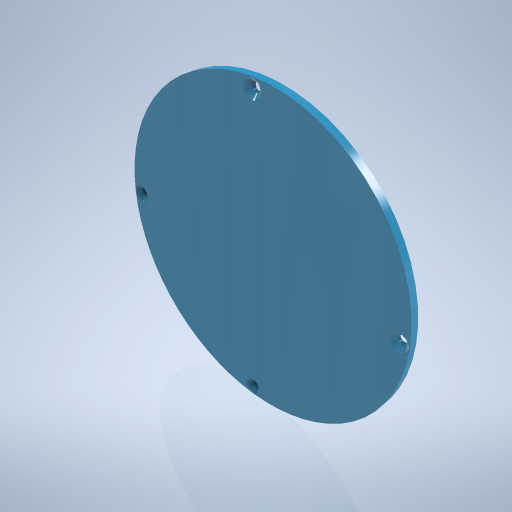
# Autodesk Inventor part: plate
Saved by Autodesk Inventor 2024.2 (Build 282272000, 272)
## iProperties
Created: 2024-04-01
Part Number: plate
Material: Gold
Document SubType Name: Modeling
Designer: Fabri
Density: 19.3 g/cm^3
Appearance: Himmelblau - dunkel
Author: Fabri
Autodesk Inventor part; units mm, degrees
ref_plane "YZ Plane" through (0, 0, 0) normal (1, 0, 0) x (0, 1, 0)
ref_plane "XZ Plane" through (0, 0, 0) normal (0, 1, 0) x (-1, 0, 0)
ref_plane "XY Plane" through (0, 0, 0) normal (0, 0, 1) x (1, 0, 0)
sketch "Skizze1" plane through (0, 0, 0) normal (0, 0, 1) x (1, 0, 0)
  line L0 (0, 0) -> (0, 15)
  line L1 (0, 2.5) -> (-9, 2.5)
  line L2 (-9, 2.5) -> (-9.567, 1.5179)
  arc A0 (-10.433, 1.5179) -> (-9.567, 1.5179) centre (-10, 1.7679) ccw
  line L3 (-10.433, 1.5179) -> (-11, 2.5)
  line L4 (-11, 2.5) -> (-12, 2.5)
  line L5 (-12, 2.5) -> (-12.567, 1.5179)
  arc A1 (-13.433, 1.5179) -> (-12.567, 1.5179) centre (-13, 1.7679) ccw
  line L6 (-13.433, 1.5179) -> (-14, 2.5)
  line L7 (-10, 1.7679) -> (-10, 5.291) construction
  line L8 (-14, 2.5) -> (-15, 2.5)
  line L9 (-15, 2.5) -> (-15.567, 1.5179)
  arc A2 (-16.433, 1.5179) -> (-15.567, 1.5179) centre (-16, 1.7679) ccw
  line L10 (-16.433, 1.5179) -> (-17, 2.5)
  line L11 (-17, 2.5) -> (-18, 2.5)
  line L12 (-18, 2.5) -> (-18.567, 1.5179)
  arc A3 (-19.433, 1.5179) -> (-18.567, 1.5179) centre (-19, 1.7679) ccw
  line L13 (-19.433, 1.5179) -> (-20, 2.5)
  line L14 (-20, 2.5) -> (-21, 2.5)
  line L15 (-21, 2.5) -> (-21.567, 1.5179)
  arc A4 (-22.433, 1.5179) -> (-21.567, 1.5179) centre (-22, 1.7679) ccw
  line L16 (-22.433, 1.5179) -> (-23, 2.5)
  line L17 (-23, 2.5) -> (-24, 2.5)
  line L18 (-24, 2.5) -> (-24.567, 1.5179)
  arc A5 (-25.433, 1.5179) -> (-24.567, 1.5179) centre (-25, 1.7679) ccw
  line L19 (-25.433, 1.5179) -> (-26, 2.5)
  line L20 (-26, 2.5) -> (-27, 2.5)
  line L21 (-27, 2.5) -> (-27.567, 1.5179)
  arc A6 (-28.433, 1.5179) -> (-27.567, 1.5179) centre (-28, 1.7679) ccw
  line L22 (-28.433, 1.5179) -> (-29, 2.5)
  line L23 (-29, 2.5) -> (-30, 2.5)
  line L24 (-30, 2.5) -> (-30.567, 1.5179)
  arc A7 (-31.433, 1.5179) -> (-30.567, 1.5179) centre (-31, 1.7679) ccw
  line L25 (-31.433, 1.5179) -> (-32, 2.5)
  line L26 (-32, 2.5) -> (-33, 2.5)
  line L27 (-33, 2.5) -> (-33.567, 1.5179)
  arc A8 (-34.433, 1.5179) -> (-33.567, 1.5179) centre (-34, 1.7679) ccw
  line L28 (-34.433, 1.5179) -> (-35, 2.5)
  line L29 (-35, 2.5) -> (-36, 2.5)
  line L30 (-36, 2.5) -> (-36.567, 1.5179)
  arc A9 (-37.433, 1.5179) -> (-36.567, 1.5179) centre (-37, 1.7679) ccw
  line L31 (-37.433, 1.5179) -> (-38, 2.5)
  line L32 (-38, 2.5) -> (-50, 2.5)
  line L33 (-50, 2.5) -> (-50, 0)
  line L34 (-50, 0) -> (0, 0)
  line L35 (0, 2.5) -> (0, 0)
  dimension "d0" = 15
  dimension "d1" = 0.5
  dimension "d2" = 60
  dimension "d3" = 3
  dimension "d4" = 2
  dimension "d7" = 3
  dimension "d12" = 2.5
  dimension "d13" = 100
  dimension "d14" = 20
  constraints: 72 end point, 20 point on circle, 10 centre point, 10 point on line, 4 tangent, 3 horizontal, 3 horizontal alignment, 3 parallel, 3 perpendicular, 2 vertical, 1 collinear, 1 equal radius, 1 symmetric about line, 80 other
  measures "d0" distance of L0.start L0.end
  measures "d1" radius of A0
  measures "d2" angle of L2 L3
  measures "d3" distance of A1.centre L7.start
  measures "d4" distance of L4.end L6.end
  measures "d7" distance of L3.end L8.start
  measures "d12" distance of L32.end L33.end
  measures "d13" diameter of L33 L0
  measures "d14" diameter of L7.start L0
revolve "Umdrehung1" add sketch "Skizze1" angle 360 about axis through (0, 0, 0) along (0, 1, 0)
sketch "Skizze2" plane through (0, 0, 0) normal (0, 1, 0) x (1, 0, 0)
  line L0 (27.8185, 0) -> (-13.7399, 0) construction
  line L1 (0, -40.9898) -> (0, 18.567) construction
  circle A0 centre (0, 0) radius 18.567 projected
  point P0 (0, -47)
  point P1 (0, 47)
  point P2 (-47, 0)
  point P3 (47, 0)
  dimension "d16" = 94
  dimension "d17" = 94
  constraints: 4 end point, 3 vertical alignment, 2 horizontal alignment, 2 symmetric about line, 1 horizontal, 1 vertical, 1 other
  measures "d16" distance of point (0, 47) point (0, -47)
  measures "d17" distance of point (47, 0) point (-47, 0)
hole "Bohrung1" at (0, 0, 47) at (0, 0, -47) at (-47, 0, 0) at (47, 0, 0) direction (0, 1, 0) diameter 2.7 end through all countersink diameter 5.5 countersink angle 90
